Nema 14 (Autodesk Fusion 360 design; units mm, degrees)
Autodesk Fusion 360 part; units mm, degrees
sketch "Sketch1" plane through (0, 0, 0) normal (0, 0, 1) x (1, 0, 0)
  line L0 (17.5, -17.5) -> (-17.5, -17.5)
  line L1 (-17.5, -17.5) -> (-17.5, 17.5)
  line L2 (-17.5, 17.5) -> (17.5, 17.5)
  line L3 (17.5, 17.5) -> (17.5, -17.5)
  line L4 (17.5, -17.5) -> (-17.5, 17.5) construction
  line L5 (-17.5, -17.5) -> (17.5, 17.5) construction
  dimension "d1" = 35
  dimension "d2" = 35
  constraint perpendicular L0 L1
  constraint parallel L0 L2
  constraint parallel L1 L3
  constraint horizontal L0
  constraint coincident L4 origin
  constraint coincident L5 origin
  measures "d1" distance of L0.end L1.end
  measures "d2" distance of L1.end L2.end
extrude "Extrude1" add sketch "Sketch1" along normal blind 34
sketch "Sketch2" plane through (0, 0, 34) normal (0, 0, 1) x (-1, 0, 0)
  line L0 (-17.5, -17.5) -> (17.5, -17.5)
  line L1 (17.5, -17.5) -> (17.5, 17.5)
  line L2 (17.5, 17.5) -> (-17.5, 17.5)
  line L3 (-17.5, 17.5) -> (-17.5, -17.5)
  circle A0 centre (0, 0) radius 11
  line L4 (-13, 13) -> (13, 13) construction
  line L5 (13, 13) -> (13, -13) construction
  line L6 (13, -13) -> (-13, -13) construction
  line L7 (-13, -13) -> (-13, 13) construction
  line L8 (-13, 13) -> (13, -13) construction
  line L9 (13, 13) -> (-13, -13) construction
  circle A1 centre (13, -13) radius 1.5
  circle A2 centre (-13, -13) radius 1.5
  circle A3 centre (-13, 13) radius 1.5
  circle A4 centre (13, 13) radius 1.5
  dimension "d5" = 22
  dimension "d6" = 26
  dimension "d7" = 26
  dimension "d8" = 3
  dimension "d9" = 3
  dimension "d10" = 3
  dimension "d11" = 3
  constraint coincident A0.centre origin
  constraint perpendicular L4 L5
  constraint parallel L4 L6
  constraint parallel L5 L7
  constraint horizontal L4
  constraint coincident L8 A0.centre
  constraint coincident L9 A0.centre
  constraint coincident L5.end L6.start
  constraint coincident L6.end L7.start
  constraint coincident L4.start L7.end
  constraint coincident L4.end L5.start
  measures "d5" diameter of A0
  measures "d6" distance of L4.end L5.end
  measures "d7" distance of L5.end L6.end
  measures "d8" diameter of A1
  measures "d9" diameter of A2
  measures "d10" diameter of A3
  measures "d11" diameter of A4
extrude "Extrude2" cut sketch "Sketch2" against normal blind 10 contours A1 | A2 | A3 | A4
extrude "Extrude3" add sketch "Sketch2" along normal blind 2.5 contours A0
sketch "Sketch3" plane through (0, 0, 36.5) normal (0, 0, 1) x (-1, 0, 0)
  circle A0 centre (0, 0) radius 11
  circle A1 centre (0, 0) radius 2.5
  dimension "d16" = 5
  constraint concentric A0 A1
  measures "d16" diameter of A1
extrude "Extrude4" add sketch "Sketch3" along normal blind 22 contours A1
chamfer "Chamfer1" distance 0.2 angle 45 1 edges at (2.3308, 0.904, 58.5)
chamfer "Chamfer2" distance 2 angle 45 4 edges at (17.5, -17.5, 17) (-17.5, -17.5, 17) (17.5, 17.5, 17) (-17.5, 17.5, 17)
fillet "Fillet1" radius 0.5 20 faces at (17.5, -5.1667, 22.6667) (-10.9863, 0.5483, 35.6667) (16.8333, -16.1667, 11.3333) (-12.75, -12.567, 24) (-5.1667, 5.8333, 0) (11.5019, 13.0748, 27.3333) (-16.1667, 16.8333, 11.3333) (-16.8333, -16.1667, 11.3333) (16.1667, 16.8333, 11.3333) (-0.274, -15.3231, 34) (5.1667, 17.5, 22.6667) (-5.1667, -17.5, 22.6667) (-17.5, 5.1667, 22.6667) (-8.1257, 0.5465, 36.5) (13.8598, 12.9255, 24) (-14.4981, -12.9252, 27.3333) (-12.75, 13.433, 24) (13.25, -12.567, 24) (11.5019, -12.9252, 27.3333) (-14.4981, 13.0748, 27.3333)
